Autodesk Fusion 360 part; units mm, degrees
(part 8 of 23)
  arc A626 (13.2203, 51.9113) -> (13.2203, 52.2287) centre (13.2203, 52.07) ccw
  arc A627 (5.1816, 11.4173) -> (5.0292, 11.4173) centre (5.1054, 11.4173) ccw
  line L5 (12.319, 44.069) -> (13.97, 44.069)
  arc A628 (84.2253, 50.6413) -> (84.2253, 50.9588) centre (84.2253, 50.8001) ccw
  arc A629 (10.6803, 51.9113) -> (10.6803, 52.2287) centre (10.6803, 52.07) ccw
  arc A630 (80.3275, 51.5938) -> (80.3275, 51.2763) centre (80.3275, 51.4351) ccw
  line L6 (20.32, 40.64) -> (25.4, 40.64)
  arc A631 (10.1061, 41.9639) -> (10.2139, 41.8561) centre (10.16, 41.91) ccw
  arc A632 (76.9767, 52.5463) -> (76.9767, 52.8638) centre (76.9767, 52.7051) ccw
  arc A633 (25.4, 40.5638) -> (25.4, 40.7162) centre (25.4, 40.64) ccw
  arc A634 (14.7197, 52.2287) -> (14.7197, 51.9113) centre (14.7197, 52.07) ccw
  arc A635 (20.32, 40.7162) -> (20.32, 40.5638) centre (20.32, 40.64) ccw
  arc A636 (4.6355, 51.2763) -> (4.6355, 51.5938) centre (4.6355, 51.4351) ccw
  arc A637 (74.93, 50.9588) -> (74.93, 50.6413) centre (74.93, 50.8001) ccw
  arc A638 (59.7335, 50.6413) -> (59.7335, 50.9588) centre (59.7335, 50.8001) ccw
  arc A639 (17.2597, 52.2287) -> (17.2597, 51.9113) centre (17.2597, 52.07) ccw
  arc A640 (8.0326, 51.5938) -> (8.0326, 51.2763) centre (8.0326, 51.4351) ccw
  arc A641 (22.3397, 52.2287) -> (22.3397, 51.9113) centre (22.3397, 52.07) ccw
  arc A642 (7.9863, 52.8638) -> (7.9863, 52.5463) centre (7.9863, 52.7051) ccw
  arc A643 (4.0005, 51.5938) -> (4.0005, 51.2763) centre (4.0005, 51.4351) ccw
  arc A644 (80.9625, 50.6413) -> (80.9625, 50.9588) centre (80.9625, 50.8001) ccw
  arc A645 (57.1065, 50.9588) -> (57.1065, 50.6413) centre (57.1065, 50.8001) ccw
  arc A646 (23.1009, 51.5938) -> (23.1009, 51.2763) centre (23.1009, 51.4351) ccw
  arc A647 (62.1865, 50.9588) -> (62.1865, 50.6413) centre (62.1865, 50.8001) ccw
  arc A648 (80.3275, 51.9113) -> (80.3275, 52.2287) centre (80.3275, 52.07) ccw
  arc A649 (59.6465, 50.9588) -> (59.6465, 50.6413) centre (59.6465, 50.8001) ccw
  arc A650 (75.5997, 50.9588) -> (75.5997, 50.6413) centre (75.5997, 50.8001) ccw
  arc A651 (19.05, 51.2763) -> (19.05, 51.5938) centre (19.05, 51.4351) ccw
  arc A652 (80.3275, 50.9588) -> (80.3275, 50.6413) centre (80.3275, 50.8001) ccw
  arc A653 (77.0766, 50.6413) -> (77.0766, 50.9588) centre (77.0766, 50.8001) ccw
  arc A654 (57.1935, 50.6413) -> (57.1935, 50.9588) centre (57.1935, 50.8001) ccw
  line L7 (25.4, 40.64) -> (26.67, 41.91)
  line L8 (5.1054, 6.3754) -> (5.1054, 11.4173)
  arc A655 (8.128, 41.9862) -> (8.128, 41.8338) centre (8.128, 41.91) ccw
  arc A656 (71.755, 10.2362) -> (71.755, 10.0838) centre (71.755, 10.16) ccw
  arc A657 (13.9161, 6.2961) -> (14.0239, 6.4039) centre (13.97, 6.35) ccw
  arc A658 (81.0545, 21.3645) -> (80.9467, 21.2567) centre (81.0006, 21.3106) ccw
  arc A659 (80.7212, 21.2344) -> (80.7212, 21.3868) centre (80.7212, 21.3106) ccw
  arc A660 (79.5559, 14.6781) -> (79.4481, 14.7859) centre (79.502, 14.732) ccw
  arc A661 (81.661, 14.6558) -> (81.661, 14.8082) centre (81.661, 14.732) ccw
  arc A662 (12.319, 44.1452) -> (12.319, 43.9928) centre (12.319, 44.069) ccw
  arc A663 (6.088, 55.4038) -> (6.088, 55.0863) centre (6.088, 55.2451) ccw
  arc A664 (5.1593, 6.3215) -> (5.0515, 6.4293) centre (5.1054, 6.3754) ccw
  line L9 (10.16, 41.91) -> (12.319, 44.069)
  arc A665 (26.7462, 38.1) -> (26.5938, 38.1) centre (26.67, 38.1) ccw
  line L10 (82.55, 19.7612) -> (81.0006, 21.3106)
  arc A666 (5.0134, 6.3912) -> (5.1212, 6.2834) centre (5.0673, 6.3373) ccw
  line L11 (5.0673, 6.3373) -> (5.1054, 6.3754)
  arc A667 (78.875, 55.0863) -> (78.875, 55.4038) centre (78.875, 55.2451) ccw
  line L12 (8.128, 41.91) -> (10.16, 41.91)
  arc A668 (82.4738, 15.621) -> (82.6262, 15.621) centre (82.55, 15.621) ccw
  line L13 (5.08, 15.24) -> (7.62, 15.24)
  arc A669 (82.6039, 15.5671) -> (82.4961, 15.6749) centre (82.55, 15.621) ccw
  arc A670 (25.3461, 40.6939) -> (25.4539, 40.5861) centre (25.4, 40.64) ccw
  arc A671 (81.6071, 14.7859) -> (81.7149, 14.6781) centre (81.661, 14.732) ccw
  line L14 (74.2188, 21.3106) -> (80.7212, 21.3106)
  arc A672 (12.3729, 44.0151) -> (12.2651, 44.1229) centre (12.319, 44.069) ccw
  arc A673 (82.4961, 19.7073) -> (82.6039, 19.8151) centre (82.55, 19.7612) ccw
  arc A674 (80.9467, 21.3645) -> (81.0545, 21.2567) centre (81.0006, 21.3106) ccw
  arc A675 (82.6262, 25.4) -> (82.4738, 25.4) centre (82.55, 25.4) ccw
  arc A676 (5.0292, 6.3754) -> (5.1816, 6.3754) centre (5.1054, 6.3754) ccw
  arc A677 (81.0006, 21.2344) -> (81.0006, 21.3868) centre (81.0006, 21.3106) ccw
  arc A678 (13.97, 43.9928) -> (13.97, 44.1452) centre (13.97, 44.069) ccw
  arc A679 (26.5938, 34.29) -> (26.7462, 34.29) centre (26.67, 34.29) ccw
  arc A680 (5.08, 15.3162) -> (5.08, 15.1638) centre (5.08, 15.24) ccw
  line L15 (82.55, 15.621) -> (82.55, 19.7612)
  line L16 (45.72, 17.78) -> (49.53, 13.97)
  arc A681 (11.4839, 8.9439) -> (11.3761, 8.8361) centre (11.43, 8.89) ccw
  arc A682 (82.4738, 22.86) -> (82.6262, 22.86) centre (82.55, 22.86) ccw
  line L17 (41.91, 25.4) -> (41.91, 24.892)
  arc A683 (71.7011, 10.1061) -> (71.8089, 10.2139) centre (71.755, 10.16) ccw
  arc A684 (67.9989, 14.0239) -> (67.8911, 13.9161) centre (67.945, 13.97) ccw
  arc A685 (74.2188, 21.3868) -> (74.2188, 21.2344) centre (74.2188, 21.3106) ccw
  arc A686 (80.7212, 21.3868) -> (80.7212, 21.2344) centre (80.7212, 21.3106) ccw
  arc A687 (82.6262, 19.7612) -> (82.4738, 19.7612) centre (82.55, 19.7612) ccw
  arc A688 (82.6039, 22.8061) -> (82.4961, 22.9139) centre (82.55, 22.86) ccw
  line L18 (81.0006, 21.3106) -> (82.55, 22.86)
  line L19 (74.93, 10.16) -> (79.502, 14.732)
  line L20 (79.502, 14.732) -> (81.661, 14.732)
  arc A689 (11.5062, 11.43) -> (11.3538, 11.43) centre (11.43, 11.43) ccw
  line L21 (7.62, 15.24) -> (11.43, 11.43)
  arc A690 (7.62, 15.1638) -> (7.62, 15.3162) centre (7.62, 15.24) ccw
  arc A691 (45.6438, 17.78) -> (45.7962, 17.78) centre (45.72, 17.78) ccw
  arc A692 (45.7962, 21.082) -> (45.6438, 21.082) centre (45.72, 21.082) ccw
  line L22 (25.4, 49.53) -> (21.59, 49.53)
  line L23 (82.55, 22.86) -> (82.55, 25.4)
  line L24 (49.53, 13.97) -> (67.945, 13.97)
  arc A693 (41.8338, 24.892) -> (41.9862, 24.892) centre (41.91, 24.892) ccw
  line L25 (67.945, 13.97) -> (71.755, 10.16)
  line L26 (11.43, 11.43) -> (11.43, 8.89)
  arc A694 (49.53, 14.0462) -> (49.53, 13.8938) centre (49.53, 13.97) ccw
  arc A695 (74.93, 10.0838) -> (74.93, 10.2362) centre (74.93, 10.16) ccw
  arc A696 (41.9639, 24.9459) -> (41.8561, 24.8381) centre (41.91, 24.892) ccw
  line L27 (11.43, 8.89) -> (13.97, 6.35)
  line L28 (45.72, 21.082) -> (45.72, 17.78)
  arc A697 (25.4, 49.3713) -> (25.4, 49.6887) centre (25.4, 49.53) ccw
  arc A698 (67.945, 13.8938) -> (67.945, 14.0462) centre (67.945, 13.97) ccw
  arc A699 (41.9862, 25.4) -> (41.8338, 25.4) centre (41.91, 25.4) ccw
  arc A700 (7.6739, 15.2939) -> (7.5661, 15.1861) centre (7.62, 15.24) ccw
  arc A701 (45.7739, 17.8339) -> (45.6661, 17.7261) centre (45.72, 17.78) ccw
  arc A702 (49.4761, 13.9161) -> (49.5839, 14.0239) centre (49.53, 13.97) ccw
  line L29 (71.755, 10.16) -> (74.93, 10.16)
  line L30 (45.72, 21.082) -> (41.91, 24.892)
  arc A703 (11.3538, 8.89) -> (11.5062, 8.89) centre (11.43, 8.89) ccw
  line L31 (81.661, 14.732) -> (82.55, 15.621)
  line L32 (80.7212, 21.3106) -> (81.0006, 21.3106)
  line L33 (26.67, 38.1) -> (26.67, 34.29)
  arc A704 (26.7239, 41.8561) -> (26.6161, 41.9639) centre (26.67, 41.91) ccw
  arc A705 (79.502, 14.8082) -> (79.502, 14.6558) centre (79.502, 14.732) ccw
  arc A706 (45.6661, 21.0281) -> (45.7739, 21.1359) centre (45.72, 21.082) ccw
  arc A707 (11.3761, 11.3761) -> (11.4839, 11.4839) centre (11.43, 11.43) ccw
  arc A708 (74.8761, 10.2139) -> (74.9839, 10.1061) centre (74.93, 10.16) ccw
  arc A709 (21.59, 49.6887) -> (21.59, 49.3713) centre (21.59, 49.53) ccw
  arc A710 (57.73, 2.7178) -> (57.73, 2.7686) centre (57.73, 2.7432) ccw
  arc A711 (55.827, 1.5494) -> (55.827, 1.6002) centre (55.827, 1.5748) ccw
  arc A712 (56.3204, 2.7512) -> (56.2722, 2.7352) centre (56.2963, 2.7432) ccw
  arc A713 (54.5067, 2.7178) -> (54.5067, 2.7686) centre (54.5067, 2.7432) ccw
  arc A714 (46.887, 2.4186) -> (46.9378, 2.4186) centre (46.9124, 2.4186) ccw
  arc A715 (59.4219, 1.8994) -> (59.4727, 1.8994) centre (59.4473, 1.8994) ccw
  line L34 (53.2144, 2.0616) -> (53.5715, 2.2564)
  arc A716 (48.3304, 2.0827) -> (48.285, 2.1054) centre (48.3077, 2.0941) ccw
  arc A717 (53.2023, 2.0839) -> (53.2266, 2.0393) centre (53.2145, 2.0616) ccw
  arc A718 (48.6718, 1.5748) -> (48.7226, 1.5748) centre (48.6972, 1.5748) ccw
  line L35 (49.8306, 1.5748) -> (49.8306, 2.7432)
  arc A719 (53.4416, 2.7686) -> (53.4416, 2.7178) centre (53.4416, 2.7432) ccw
  arc A720 (57.73, 1.5494) -> (57.73, 1.6002) centre (57.73, 1.5748) ccw
  arc A721 (58.2535, 2.7432) -> (58.2027, 2.7432) centre (58.2281, 2.7432) ccw
  line L36 (58.8772, 1.5748) -> (58.8772, 2.7432)
  arc A722 (54.8059, 1.5748) -> (54.8567, 1.5748) centre (54.8313, 1.5748) ccw
  arc A723 (55.3077, 2.7686) -> (55.3077, 2.7178) centre (55.3077, 2.7432) ccw
  arc A724 (53.7013, 2.4836) -> (53.4416, 2.7432) centre (53.4416, 2.4835) ccw
  line L37 (55.827, 2.7432) -> (55.3077, 2.7432)
  arc A725 (54.8313, 2.7178) -> (54.8313, 2.7686) centre (54.8313, 2.7432) ccw
  line L38 (54.8313, 1.5748) -> (54.8313, 2.7432)
  arc A726 (49.8052, 1.5748) -> (49.856, 1.5748) centre (49.8306, 1.5748) ccw
  arc A727 (53.6759, 2.4836) -> (53.7267, 2.4836) centre (53.7013, 2.4836) ccw
  arc A728 (59.4727, 2.7432) -> (59.4219, 2.7432) centre (59.4473, 2.7432) ccw
  arc A729 (57.4703, 2.7686) -> (57.4703, 2.7178) centre (57.4703, 2.7432) ccw
  arc A730 (54.5067, 2.7686) -> (54.5067, 2.7178) centre (54.5067, 2.7432) ccw
  arc A731 (46.9124, 1.8994) -> (47.5615, 1.8994) centre (47.237, 1.8994) ccw
  arc A732 (46.9378, 1.8994) -> (46.887, 1.8994) centre (46.9124, 1.8994) ccw
  arc A733 (52.0122, 1.8923) -> (52.0122, 1.8415) centre (52.0122, 1.8669) ccw
  arc A734 (55.827, 2.7178) -> (55.827, 2.7686) centre (55.827, 2.7432) ccw
  arc A735 (53.4416, 2.7432) -> (53.1495, 2.6458) centre (53.4416, 2.2564) ccw
  arc A736 (58.8518, 1.5748) -> (58.9026, 1.5748) centre (58.8772, 1.5748) ccw
  line L39 (54.8313, 2.7432) -> (54.5067, 2.7432)
  arc A737 (54.5067, 2.7432) -> (54.5067, 2.0941) centre (54.5067, 2.4186) ccw
  arc A738 (52.5964, 1.8415) -> (52.5964, 1.8923) centre (52.5964, 1.8669) ccw
  arc A739 (54.5067, 2.0687) -> (54.5067, 2.1195) centre (54.5067, 2.0941) ccw
  arc A740 (49.506, 2.7178) -> (49.506, 2.7686) centre (49.506, 2.7432) ccw
  line L40 (57.6002, 2.7432) -> (57.6002, 1.5748)
  arc A741 (51.8907, 1.5828) -> (51.9389, 1.5668) centre (51.9148, 1.5748) ccw
  arc A742 (53.7518, 1.7192) -> (53.7157, 1.755) centre (53.7338, 1.7371) ccw
  arc A743 (50.9262, 1.6002) -> (50.9262, 1.5494) centre (50.9262, 1.5748) ccw
  line L41 (49.506, 2.0941) -> (49.8306, 2.0941)
  arc A744 (58.8994, 2.7309) -> (58.855, 2.7555) centre (58.8772, 2.7432) ccw
  arc A745 (46.887, 1.8994) -> (46.9378, 1.8994) centre (46.9124, 1.8994) ccw
  arc A746 (49.8306, 2.0687) -> (49.8306, 2.1195) centre (49.8306, 2.0941) ccw
  arc A747 (55.8016, 1.5748) -> (55.8524, 1.5748) centre (55.827, 1.5748) ccw
  line L42 (51.4455, 2.7432) -> (51.4455, 1.5748)
  line L43 (51.4455, 1.5748) -> (50.9262, 1.5748)
  arc A748 (58.2059, 1.5871) -> (58.2503, 1.5625) centre (58.2281, 1.5748) ccw
  arc A749 (53.1343, 2.6662) -> (53.1648, 2.6255) centre (53.1496, 2.6458) ccw
  line L44 (57.73, 2.7432) -> (57.4703, 2.7432)
  arc A750 (57.6256, 2.7432) -> (57.5748, 2.7432) centre (57.6002, 2.7432) ccw
  arc A751 (53.5715, 2.2564) -> (53.7013, 2.4836) centre (53.4376, 2.4836) ccw
  arc A752 (52.3284, 2.7512) -> (52.2802, 2.7352) centre (52.3043, 2.7432) ccw
  arc A753 (49.506, 2.0687) -> (49.506, 2.1195) centre (49.506, 2.0941) ccw
  arc A754 (49.856, 2.7432) -> (49.8052, 2.7432) centre (49.8306, 2.7432) ccw
  arc A755 (48.7226, 2.7432) -> (48.6718, 2.7432) centre (48.6972, 2.7432) ccw
  line L45 (52.6937, 1.5748) -> (52.3043, 2.7432)
  arc A756 (54.8567, 2.7432) -> (54.8059, 2.7432) centre (54.8313, 2.7432) ccw
  arc A757 (48.6972, 2.7178) -> (48.6972, 2.7686) centre (48.6972, 2.7432) ccw
  arc A758 (53.2273, 2.0397) -> (53.2015, 2.0835) centre (53.2144, 2.0616) ccw
  arc A759 (47.5869, 2.4186) -> (47.5361, 2.4186) centre (47.5615, 2.4186) ccw
  arc A760 (49.8306, 2.7178) -> (49.8306, 2.7686) centre (49.8306, 2.7432) ccw
  arc A761 (48.3726, 2.7432) -> (48.3726, 2.0941) centre (48.3726, 2.4186) ccw
  line L46 (48.6972, 2.7432) -> (48.3726, 2.7432)
  line L47 (49.8306, 2.7432) -> (49.506, 2.7432)
  arc A762 (49.506, 2.7686) -> (49.506, 2.7178) centre (49.506, 2.7432) ccw
  arc A763 (48.3726, 2.7178) -> (48.3726, 2.7686) centre (48.3726, 2.7432) ccw
  line L48 (46.9124, 2.4186) -> (46.9124, 1.8994)
  arc A764 (53.2144, 2.0616) -> (53.0846, 1.8344) centre (53.3483, 1.8344) ccw
  arc A765 (53.7267, 2.4836) -> (53.6759, 2.4836) centre (53.7013, 2.4836) ccw
  arc A766 (52.3284, 2.7352) -> (52.2802, 2.7512) centre (52.3043, 2.7432) ccw
  arc A767 (48.0253, 1.5862) -> (48.0708, 1.5634) centre (48.0481, 1.5748) ccw
  line L49 (48.0481, 1.5748) -> (48.3077, 2.0941)
  line L50 (48.6972, 1.5748) -> (48.6972, 2.7432)
  arc A768 (46.9378, 2.4186) -> (46.887, 2.4186) centre (46.9124, 2.4186) ccw
  arc A769 (48.3726, 2.1195) -> (48.3726, 2.0687) centre (48.3726, 2.0941) ccw
  arc A770 (44.3715, 2.7178) -> (44.3715, 2.7686) centre (44.3715, 2.7432) ccw
  arc A771 (43.7515, 2.7178) -> (43.7515, 2.7686) centre (43.7515, 2.7432) ccw
  arc A772 (40.9609, 2.4836) -> (40.9101, 2.4836) centre (40.9355, 2.4836) ccw
  arc A773 (40.4162, 1.6002) -> (40.4162, 1.5494) centre (40.4162, 1.5748) ccw
  arc A774 (41.6956, 2.0687) -> (41.6956, 2.1195) centre (41.6956, 2.0941) ccw
  line L51 (40.9355, 1.8344) -> (40.9355, 2.4836)
  arc A775 (40.9101, 1.8344) -> (40.9609, 1.8344) centre (40.9355, 1.8344) ccw
  arc A776 (47.5615, 2.4186) -> (46.9124, 2.4186) centre (47.237, 2.4186) ccw
  arc A777 (53.5836, 2.2341) -> (53.5593, 2.2787) centre (53.5714, 2.2564) ccw
  line L52 (48.3726, 2.0941) -> (48.6972, 2.0941)
  arc A778 (42.0201, 2.7178) -> (42.0201, 2.7686) centre (42.0201, 2.7432) ccw
  arc A779 (42.0455, 2.7432) -> (41.9947, 2.7432) centre (42.0201, 2.7432) ccw
  arc A780 (48.3726, 2.7686) -> (48.3726, 2.7178) centre (48.3726, 2.7432) ccw
  line L53 (47.5615, 1.8994) -> (47.5615, 2.4186)
  arc A781 (51.4455, 1.5494) -> (51.4455, 1.6002) centre (51.4455, 1.5748) ccw
  arc A782 (47.5361, 2.4186) -> (47.5869, 2.4186) centre (47.5615, 2.4186) ccw
  arc A783 (40.9609, 1.8344) -> (40.9101, 1.8344) centre (40.9355, 1.8344) ccw
  line L54 (45.5781, 2.7432) -> (45.0588, 2.7432)
  arc A784 (46.1458, 1.8344) -> (46.4054, 1.5748) centre (46.4054, 1.8344) ccw
  arc A785 (47.5361, 1.8994) -> (47.5869, 1.8994) centre (47.5615, 1.8994) ccw
  arc A786 (41.6956, 2.7178) -> (41.6956, 2.7686) centre (41.6956, 2.7432) ccw
  arc A787 (45.5781, 2.7178) -> (45.5781, 2.7686) centre (45.5781, 2.7432) ccw
  arc A788 (44.3715, 1.5494) -> (44.3715, 1.6002) centre (44.3715, 1.5748) ccw
  arc A789 (49.506, 2.1195) -> (49.506, 2.0687) centre (49.506, 2.0941) ccw
  arc A790 (44.6566, 2.4836) -> (44.6058, 2.4836) centre (44.6312, 2.4836) ccw
  arc A791 (41.9947, 1.5748) -> (42.0455, 1.5748) centre (42.0201, 1.5748) ccw
  arc A792 (53.4416, 2.7178) -> (53.4416, 2.7686) centre (53.4416, 2.7432) ccw
  arc A793 (51.4709, 2.7432) -> (51.4201, 2.7432) centre (51.4455, 2.7432) ccw
  arc A794 (52.6696, 1.5668) -> (52.7178, 1.5828) centre (52.6937, 1.5748) ccw
  arc A795 (51.4201, 1.5748) -> (51.4709, 1.5748) centre (51.4455, 1.5748) ccw
  line L55 (52.0122, 1.8669) -> (52.5964, 1.8669)
  arc A796 (48.6972, 2.0687) -> (48.6972, 2.1195) centre (48.6972, 2.0941) ccw
  line L56 (52.3043, 2.7432) -> (51.9148, 1.5748)
  arc A797 (53.0592, 1.8344) -> (53.11, 1.8344) centre (53.0846, 1.8344) ccw
  arc A798 (43.4524, 2.7432) -> (43.4016, 2.7432) centre (43.427, 2.7432) ccw
  arc A799 (44.6566, 1.8344) -> (44.6058, 1.8344) centre (44.6312, 1.8344) ccw
  arc A800 (53.5586, 2.2782) -> (53.5843, 2.2345) centre (53.5714, 2.2564) ccw
  arc A801 (46.1204, 1.8344) -> (46.1712, 1.8344) centre (46.1458, 1.8344) ccw
  line L57 (44.6312, 1.8344) -> (44.6312, 2.4836)
  arc A802 (49.506, 2.7432) -> (49.506, 2.0941) centre (49.506, 2.4186) ccw
  arc A803 (45.0588, 2.7686) -> (45.0588, 2.7178) centre (45.0588, 2.7432) ccw
  arc A804 (45.5781, 1.5494) -> (45.5781, 1.6002) centre (45.5781, 1.5748) ccw
  arc A805 (48.3726, 2.0687) -> (48.3726, 2.1195) centre (48.3726, 2.0941) ccw
  line L58 (42.0201, 1.5748) -> (42.0201, 2.7432)
  arc A806 (44.6058, 2.4836) -> (44.6566, 2.4836) centre (44.6312, 2.4836) ccw
  line L59 (45.5781, 2.2239) -> (45.1886, 2.2239)
  line L60 (40.4162, 1.5748) -> (40.6758, 1.5748)
  arc A807 (43.4016, 1.5748) -> (43.4524, 1.5748) centre (43.427, 1.5748) ccw
  arc A808 (36.7595, 1.5494) -> (36.7595, 1.6002) centre (36.7595, 1.5748) ccw
  arc A809 (36.6946, 2.7432) -> (36.6946, 2.2239) centre (36.6946, 2.4836) ccw
  arc A810 (44.1119, 1.6002) -> (44.1119, 1.5494) centre (44.1119, 1.5748) ccw
  arc A811 (40.9355, 2.4836) -> (40.6758, 2.7432) centre (40.6758, 2.4835) ccw
  arc A812 (46.5352, 1.5494) -> (46.5352, 1.6002) centre (46.5352, 1.5748) ccw
  arc A813 (39.6001, 2.1985) -> (39.6001, 2.2493) centre (39.6001, 2.2239) ccw
  arc A814 (36.6946, 2.7178) -> (36.6946, 2.7686) centre (36.6946, 2.7432) ccw
  arc A815 (39.6001, 2.1985) -> (39.6001, 2.2493) centre (39.6001, 2.2239) ccw
  arc A816 (40.6758, 1.6002) -> (40.6758, 1.5494) centre (40.6758, 1.5748) ccw
  line L61 (45.0588, 1.5748) -> (45.5781, 1.5748)
  arc A817 (43.1024, 2.7686) -> (43.1024, 2.7178) centre (43.1024, 2.7432) ccw
  arc A818 (45.5527, 1.5748) -> (45.6035, 1.5748) centre (45.5781, 1.5748) ccw
  arc A819 (39.9246, 2.7178) -> (39.9246, 2.7686) centre (39.9246, 2.7432) ccw
  arc A820 (37.084, 1.5494) -> (37.084, 1.6002) centre (37.084, 1.5748) ccw
  line L62 (41.6956, 2.0941) -> (42.0201, 2.0941)
  arc A821 (41.6956, 2.1195) -> (41.6956, 2.0687) centre (41.6956, 2.0941) ccw
  arc A822 (46.1712, 1.8344) -> (46.1204, 1.8344) centre (46.1458, 1.8344) ccw
  arc A823 (41.6956, 2.7432) -> (41.6956, 2.0941) centre (41.6956, 2.4186) ccw
  arc A824 (39.6001, 1.6002) -> (39.6001, 1.5494) centre (39.6001, 1.5748) ccw
  arc A825 (41.6956, 2.7686) -> (41.6956, 2.7178) centre (41.6956, 2.7432) ccw
  line L63 (46.4054, 1.5748) -> (46.5352, 1.5748)
  arc A826 (46.4054, 1.5494) -> (46.4054, 1.6002) centre (46.4054, 1.5748) ccw
  line L64 (43.7515, 2.7432) -> (43.1024, 2.7432)
  line L65 (44.1119, 1.5748) -> (44.3715, 1.5748)
  arc A827 (40.4162, 2.7686) -> (40.4162, 2.7178) centre (40.4162, 2.7432) ccw
  arc A828 (44.6312, 2.4836) -> (44.3715, 2.7432) centre (44.3715, 2.4835) ccw
  arc A829 (46.4054, 1.6002) -> (46.4054, 1.5494) centre (46.4054, 1.5748) ccw
  arc A830 (40.9101, 2.4836) -> (40.9609, 2.4836) centre (40.9355, 2.4836) ccw
  arc A831 (36.6946, 2.1985) -> (36.6946, 2.2493) centre (36.6946, 2.2239) ccw
  arc A832 (45.1886, 2.2493) -> (45.1886, 2.1985) centre (45.1886, 2.2239) ccw
  line L66 (46.1458, 2.7432) -> (46.1458, 1.8344)
  arc A833 (44.3715, 1.5748) -> (44.6312, 1.8344) centre (44.3715, 1.8345) ccw
  arc A834 (45.0588, 1.6002) -> (45.0588, 1.5494) centre (45.0588, 1.5748) ccw
  line L67 (44.3715, 2.7432) -> (44.1119, 2.7432)
  line L68 (45.5781, 1.5748) -> (45.5781, 2.7432)
  arc A835 (45.5781, 2.1985) -> (45.5781, 2.2493) centre (45.5781, 2.2239) ccw
  arc A836 (39.6001, 2.2239) -> (39.6001, 1.5748) centre (39.6001, 1.8994) ccw
  arc A837 (44.3715, 2.7686) -> (44.3715, 2.7178) centre (44.3715, 2.7432) ccw
  arc A838 (44.6058, 1.8344) -> (44.6566, 1.8344) centre (44.6312, 1.8344) ccw
  line L69 (37.9025, 1.5748) -> (37.513, 2.7432)
  arc A839 (36.9542, 2.1985) -> (36.9542, 2.2493) centre (36.9542, 2.2239) ccw
  arc A840 (36.6946, 2.7686) -> (36.6946, 2.7178) centre (36.6946, 2.7432) ccw
  line L70 (39.9246, 1.5748) -> (39.9246, 2.7432)
  arc A841 (40.6758, 2.7686) -> (40.6758, 2.7178) centre (40.6758, 2.7432) ccw
  arc A842 (42.0201, 2.0687) -> (42.0201, 2.1195) centre (42.0201, 2.0941) ccw
  line L71 (42.0201, 2.7432) -> (41.6956, 2.7432)
  arc A843 (38.3161, 2.7352) -> (38.2679, 2.7512) centre (38.292, 2.7432) ccw
  arc A844 (47.5869, 1.8994) -> (47.5361, 1.8994) centre (47.5615, 1.8994) ccw
  arc A845 (45.6035, 2.7432) -> (45.5527, 2.7432) centre (45.5781, 2.7432) ccw
  arc A846 (40.6758, 1.5748) -> (40.9355, 1.8344) centre (40.6758, 1.8345) ccw
  arc A847 (44.3715, 1.6002) -> (44.3715, 1.5494) centre (44.3715, 1.5748) ccw
  arc A848 (40.6758, 1.5494) -> (40.6758, 1.6002) centre (40.6758, 1.5748) ccw
  line L72 (43.427, 1.5748) -> (43.427, 2.7432)
  arc A849 (46.1712, 2.7432) -> (46.1204, 2.7432) centre (46.1458, 2.7432) ccw
  arc A850 (44.1119, 2.7686) -> (44.1119, 2.7178) centre (44.1119, 2.7432) ccw
  arc A851 (39.6001, 2.7178) -> (39.6001, 2.7686) centre (39.6001, 2.7432) ccw
  arc A852 (39.6001, 1.5494) -> (39.6001, 1.6002) centre (39.6001, 1.5748) ccw
  arc A853 (48.8132, 13.5283) -> (48.5887, 13.3038) centre (48.701, 13.416) ccw
  arc A854 (43.3224, 25.6494) -> (43.0049, 25.6494) centre (43.1637, 25.6494) ccw
  line L73 (40.8472, 24.6898) -> (40.9976, 24.5394)
  arc A855 (39.6001, 2.2493) -> (39.6001, 2.1985) centre (39.6001, 2.2239) ccw
  arc A856 (48.8638, 13.0287) -> (49.0883, 13.2532) centre (48.9761, 13.1409) ccw
  arc A857 (42.7324, 26.5751) -> (42.5079, 26.3506) centre (42.6201, 26.4629) ccw
  arc A858 (44.6298, 20.5647) -> (44.8544, 20.7892) centre (44.7421, 20.677) ccw
  line L74 (40.8472, 26.1102) -> (40.6563, 25.6494)
  arc A859 (39.9246, 1.5494) -> (39.9246, 1.6002) centre (39.9246, 1.5748) ccw
  arc A860 (37.084, 2.7178) -> (37.084, 2.7686) centre (37.084, 2.7432) ccw
  arc A861 (49.2747, 12.8454) -> (49.3962, 13.1388) centre (49.3355, 12.9921) ccw
  arc A862 (40.9594, 24.8021) -> (40.7349, 24.5776) centre (40.8472, 24.6898) ccw
  line L75 (48.701, 13.4161) -> (48.9761, 13.141)
  arc A863 (42.2201, 26.8004) -> (42.0986, 26.507) centre (42.1594, 26.6537) ccw
  arc A864 (42.5594, 26.3162) -> (42.6809, 26.6095) centre (42.6201, 26.4628) ccw
  line L76 (39.9246, 2.7432) -> (39.6001, 2.7432)
  line L77 (38.292, 2.7432) -> (37.9025, 1.5748)
  arc A865 (40.6758, 2.7178) -> (40.6758, 2.7686) centre (40.6758, 2.7432) ccw
  line L78 (37.084, 2.7432) -> (36.6946, 2.7432)
  arc A866 (39.8992, 1.5748) -> (39.95, 1.5748) centre (39.9246, 1.5748) ccw
  line L79 (40.6758, 2.7432) -> (40.4162, 2.7432)
  line L80 (44.7421, 20.6769) -> (44.7421, 17.5855)
  line L81 (12.3063, 34.2399) -> (12.3063, 33.5781)
  line L82 (37.084, 1.5748) -> (36.7595, 1.5748)
  line L83 (36.6946, 2.2239) -> (36.9542, 2.2239)
  arc A867 (41.1391, 26.6095) -> (41.2606, 26.3162) centre (41.1998, 26.4628) ccw
  arc A868 (41.3121, 26.3506) -> (41.0876, 26.5751) centre (41.1998, 26.4629) ccw
  line L84 (40.9976, 24.5394) -> (41.081, 24.3381)
  line L85 (39.9246, 2.2239) -> (39.6001, 2.2239)
  arc A869 (36.7595, 2.1985) -> (36.7595, 2.2493) centre (36.7595, 2.2239) ccw
  arc A870 (36.7595, 1.6002) -> (36.7595, 1.5494) centre (36.7595, 1.5748) ccw
  arc A871 (41.1442, 24.6002) -> (40.8509, 24.4787) centre (40.9976, 24.5395) ccw
  arc A872 (36.6946, 2.2493) -> (36.6946, 2.1985) centre (36.6946, 2.2239) ccw
  arc A873 (37.8784, 1.5828) -> (37.9266, 1.5668) centre (37.9025, 1.5748) ccw
  line L86 (41.1998, 26.4628) -> (40.8472, 26.1102)
  line L87 (40.6563, 25.1506) -> (40.8472, 24.6898)
  arc A874 (42.8606, 25.9979) -> (43.0851, 26.2224) centre (42.9729, 26.1102) ccw
  arc A875 (37.8784, 1.5668) -> (37.9266, 1.5828) centre (37.9025, 1.5748) ccw
  arc A876 (40.9938, 26.0494) -> (40.7005, 26.1709) centre (40.8471, 26.1102) ccw
  arc A877 (40.803, 25.2114) -> (40.5096, 25.0899) centre (40.6563, 25.1506) ccw
  arc A878 (36.7595, 2.2239) -> (36.7595, 1.5748) centre (36.7595, 1.8994) ccw
  line L88 (39.6001, 1.5748) -> (39.9246, 1.5748)
  arc A879 (48.5887, 13.3038) -> (48.8132, 13.5283) centre (48.701, 13.416) ccw
  line L89 (48.9761, 13.141) -> (49.3355, 12.9921)
  arc A880 (40.8853, 24.4272) -> (41.1098, 24.6517) centre (40.9976, 24.5395) ccw
  arc A881 (39.95, 2.7432) -> (39.8992, 2.7432) centre (39.9246, 2.7432) ccw
  arc A882 (39.9246, 2.1985) -> (39.9246, 2.2493) centre (39.9246, 2.2239) ccw
  line L90 (43.1637, 25.6494) -> (42.9728, 26.1102)
  line L91 (41.081, 24.3381) -> (41.3561, 24.063)
  arc A883 (39.6001, 2.7432) -> (39.6001, 2.2239) centre (39.6001, 2.4836) ccw
  line L92 (44.891, 17.2261) -> (48.701, 13.4161)
  arc A884 (39.6001, 2.7686) -> (39.6001, 2.7178) centre (39.6001, 2.7432) ccw
  arc A885 (43.3104, 25.0899) -> (43.017, 25.2114) centre (43.1637, 25.1507) ccw
  line L93 (44.7421, 17.5855) -> (44.891, 17.2261)
  arc A886 (37.5371, 2.7512) -> (37.4889, 2.7352) centre (37.513, 2.7432) ccw
  arc A887 (45.0032, 17.3383) -> (44.7787, 17.1138) centre (44.891, 17.226) ccw
  line L94 (43.1258, 25.0591) -> (43.1637, 25.1506)
  arc A888 (46.1617, 21.7988) -> (46.3862, 22.0233) centre (46.2739, 21.9111) ccw
  line L95 (42.6202, 26.4628) -> (42.1594, 26.6537)
  arc A889 (41.6606, 26.8124) -> (41.6606, 26.4949) centre (41.6606, 26.6536) ccw
  arc A890 (43.0049, 25.1506) -> (43.3224, 25.1506) centre (43.1637, 25.1506) ccw
  arc A891 (41.4683, 24.1752) -> (41.2438, 23.9507) centre (41.356, 24.063) ccw
  arc A892 (79.2435, 8.2232) -> (79.2435, 8.5407) centre (79.2435, 8.3819) ccw
  arc A893 (40.4976, 25.1506) -> (40.815, 25.1506) centre (40.6563, 25.1506) ccw
  arc A894 (42.9791, 25.1199) -> (43.2725, 24.9984) centre (43.1258, 25.0592) ccw
  arc A895 (41.2438, 23.9507) -> (41.4683, 24.1752) centre (41.356, 24.063) ccw
  line L96 (79.2435, 8.382) -> (75.7524, 8.382)
  line L97 (71.5605, 9.1821) -> (75.1245, 9.1821)
  arc A896 (44.5834, 17.5855) -> (44.9008, 17.5855) centre (44.7421, 17.5855) ccw
  line L98 (40.6563, 25.6494) -> (40.6563, 25.1506)
  arc A897 (43.017, 25.5886) -> (43.3104, 25.7101) centre (43.1637, 25.6493) ccw
  arc A898 (44.7443, 17.1653) -> (45.0376, 17.2868) centre (44.891, 17.226) ccw
  arc A899 (42.1594, 26.4949) -> (42.1594, 26.8124) centre (42.1594, 26.6536) ccw
  line L99 (81.1911, 11.8305) -> (81.6991, 11.3225)
  line L100 (41.3561, 24.063) -> (44.7421, 20.6769)
  arc A900 (81.1003, 9.0106) -> (81.1003, 9.3281) centre (81.1003, 9.1694) ccw
  arc A901 (80.4587, 9.0227) -> (80.3372, 9.3161) centre (80.398, 9.1694) ccw
  line L101 (49.3355, 12.9921) -> (67.5399, 12.9921)
  arc A902 (81.5404, 9.737) -> (81.8578, 9.737) centre (81.6991, 9.737) ccw
  arc A903 (81.8555, 13.5954) -> (81.8555, 13.9129) centre (81.8555, 13.7542) ccw
  arc A904 (81.0101, 9.2725) -> (81.2346, 9.048) centre (81.1223, 9.1603) ccw
  line L102 (70.926, 9.6061) -> (71.2011, 9.331)
  arc A905 (68.8686, 22.0663) -> (68.8686, 22.3838) centre (68.8686, 22.2251) ccw
  line L103 (42.9728, 26.1102) -> (42.6202, 26.4628)
  arc A906 (43.1195, 26.1709) -> (42.8262, 26.0494) centre (42.9729, 26.1102) ccw
  arc A907 (81.0324, 11.8305) -> (81.3499, 11.8305) centre (81.1912, 11.8305) ccw
  line L104 (79.7492, 8.9006) -> (79.2526, 8.4041)
  line L105 (41.6606, 26.6537) -> (41.1998, 26.4628)
  line L106 (43.1637, 25.1506) -> (43.1637, 25.6494)
  arc A908 (81.0616, 9.0136) -> (81.1831, 9.3069) centre (81.1223, 9.1602) ccw
  line L107 (81.9037, 13.7741) -> (81.1911, 13.0615)
  line L108 (42.1594, 26.6537) -> (41.6606, 26.6537)
  arc A909 (75.6058, 8.3213) -> (75.8991, 8.4427) centre (75.7525, 8.382) ccw
  arc A910 (75.3717, 9.4432) -> (75.5962, 9.2187) centre (75.484, 9.331) ccw
  arc A911 (40.7349, 26.2224) -> (40.9594, 25.9979) centre (40.8472, 26.1102) ccw
  line L109 (81.6991, 9.737) -> (81.1223, 9.1603)
  arc A912 (71.0382, 9.7183) -> (70.8137, 9.4938) centre (70.926, 9.606) ccw
  line L110 (67.5399, 12.9921) -> (70.926, 9.6061)
  arc A913 (79.1403, 8.5163) -> (79.3648, 8.2918) centre (79.2525, 8.4041) ccw
  arc A914 (82.0159, 13.6618) -> (81.7914, 13.8863) centre (81.9036, 13.774) ccw
  arc A915 (40.7005, 24.6291) -> (40.9938, 24.7506) centre (40.8471, 24.6898) ccw
  arc A916 (40.9343, 24.2773) -> (41.2276, 24.3988) centre (41.081, 24.3381) ccw
  arc A917 (44.8888, 17.6462) -> (44.5954, 17.5247) centre (44.7421, 17.5855) ccw
  arc A918 (41.7214, 26.507) -> (41.5999, 26.8004) centre (41.6606, 26.6537) ccw
  arc A919 (40.815, 25.6494) -> (40.4976, 25.6494) centre (40.6563, 25.6494) ccw
  arc A920 (41.1932, 24.4503) -> (40.9687, 24.2258) centre (41.081, 24.338) ccw
  line L111 (75.4839, 9.331) -> (79.9071, 13.7541)
  line L112 (75.7524, 8.382) -> (75.7433, 8.4041)
  arc A921 (80.0193, 13.6418) -> (79.7948, 13.8664) centre (79.907, 13.7541) ccw
  arc A922 (40.5096, 25.7101) -> (40.803, 25.5886) centre (40.6563, 25.6494) ccw
  line L113 (80.398, 9.1694) -> (79.7492, 8.9006)
  arc A923 (80.398, 9.3281) -> (80.398, 9.0106) centre (80.398, 9.1694) ccw
  arc A924 (44.9008, 20.6769) -> (44.5834, 20.6769) centre (44.7421, 20.6769) ccw
  arc A925 (67.5399, 12.8334) -> (67.5399, 13.1509) centre (67.5399, 12.9922) ccw
  line L114 (79.2526, 8.4041) -> (79.2435, 8.382)
  arc A926 (43.2381, 25.1714) -> (43.0136, 24.9469) centre (43.1258, 25.0591) ccw
  arc A927 (67.6522, 13.1044) -> (67.4277, 12.8798) centre (67.5399, 12.9921) ccw
  arc A928 (71.0888, 9.2187) -> (71.3133, 9.4432) centre (71.2011, 9.331) ccw
  line L115 (71.2011, 9.331) -> (71.5605, 9.1821)
  arc A929 (81.1611, 9.3161) -> (81.0395, 9.0227) centre (81.1003, 9.1694) ccw
  arc A930 (66.1005, 9.3891) -> (66.3938, 9.5106) centre (66.2472, 9.4498) ccw
  line L116 (81.1223, 9.1603) -> (81.1003, 9.1694)
  arc A931 (66.9999, 8.7596) -> (67.1214, 9.053) centre (67.0606, 8.9063) ccw
  line L117 (81.8555, 13.7541) -> (81.9037, 13.7741)
  line L118 (67.5594, 8.9063) -> (68.0202, 9.0972)
  arc A932 (79.0968, 8.4427) -> (79.3901, 8.3213) centre (79.2435, 8.382) ccw
  arc A933 (73.9563, 9.0227) -> (73.8348, 9.3161) centre (73.8956, 9.1694) ccw
  line L119 (68.0202, 11.2228) -> (67.5594, 11.4137)
  arc A934 (72.5944, 8.4427) -> (72.8877, 8.3213) centre (72.7411, 8.382) ccw
  line L120 (75.7433, 8.4041) -> (75.2467, 8.9006)
  arc A935 (70.8137, 9.4938) -> (71.0382, 9.7183) centre (70.926, 9.6061) ccw
  arc A936 (49.3355, 13.1509) -> (49.3355, 12.8334) centre (49.3355, 12.9922) ccw
  arc A937 (71.4997, 9.0354) -> (71.6212, 9.3288) centre (71.5605, 9.1821) ccw
  arc A938 (75.1859, 8.754) -> (75.3075, 9.0473) centre (75.2467, 8.9007) ccw
  arc A939 (75.359, 9.0129) -> (75.1344, 8.7884) centre (75.2467, 8.9006) ccw
  line L121 (75.2467, 8.9006) -> (74.5979, 9.1694)
  line L122 (66.5998, 11.2228) -> (66.2472, 10.8702)
  line L123 (66.0563, 10.4094) -> (66.0563, 9.9106)
  arc A940 (81.8114, 9.6248) -> (81.5868, 9.8493) centre (81.6991, 9.737) ccw
  arc A941 (79.6884, 9.0473) -> (79.8099, 8.754) centre (79.7492, 8.9007) ccw
  arc A942 (75.7524, 8.5407) -> (75.7524, 8.2232) centre (75.7524, 8.3819) ccw
  arc A943 (75.0638, 9.3288) -> (75.1853, 9.0354) centre (75.1245, 9.1821) ccw
  arc A944 (65.8976, 9.9106) -> (66.2151, 9.9106) centre (66.0564, 9.9106) ccw
  line L124 (79.9071, 13.7541) -> (81.8555, 13.7541)
  arc A945 (71.5605, 9.3408) -> (71.5605, 9.0234) centre (71.5605, 9.1821) ccw
  line L125 (81.1911, 13.0615) -> (81.1911, 11.8305)
  arc A946 (81.3499, 13.0615) -> (81.0324, 13.0615) centre (81.1912, 13.0615) ccw
  arc A947 (67.1214, 11.267) -> (66.9999, 11.5604) centre (67.0606, 11.4137) ccw
  arc A948 (81.7948, 13.9008) -> (81.9163, 13.6074) centre (81.8556, 13.7541) ccw
  arc A949 (81.5868, 11.2103) -> (81.8114, 11.4348) centre (81.6991, 11.3225) ccw
  line L126 (69.1454, 11.1379) -> (68.1051, 11.1379)
  arc A950 (66.2151, 10.4094) -> (65.8976, 10.4094) centre (66.0564, 10.4094) ccw
  arc A951 (72.8969, 8.3433) -> (72.6035, 8.4648) centre (72.7502, 8.4041) ccw
  line L127 (75.1245, 9.1821) -> (75.4839, 9.331)
  arc A952 (79.3993, 8.3433) -> (79.1059, 8.4648) centre (79.2526, 8.4041) ccw
  arc A953 (75.89, 8.4648) -> (75.5966, 8.3433) centre (75.7433, 8.4041) ccw
  arc A954 (71.2618, 9.4776) -> (71.1403, 9.1843) centre (71.201, 9.3309) ccw
  arc A955 (81.8578, 11.3225) -> (81.5404, 11.3225) centre (81.6991, 11.3225) ccw
  arc A956 (67.6201, 11.5604) -> (67.4986, 11.267) centre (67.5593, 11.4137) ccw
  arc A957 (49.0368, 13.2876) -> (48.9153, 12.9943) centre (48.9761, 13.141) ccw
  line L128 (81.1003, 9.1694) -> (80.398, 9.1694)
  line L129 (81.6991, 11.3225) -> (81.6991, 9.737)
  arc A958 (67.5594, 8.7476) -> (67.5594, 9.065) centre (67.5594, 8.9063) ccw
  arc A959 (67.0606, 9.065) -> (67.0606, 8.7476) centre (67.0606, 8.9063) ccw
  line L130 (69.5048, 10.989) -> (69.1454, 11.1379)
  arc A960 (74.6586, 9.3161) -> (74.5371, 9.0227) centre (74.5978, 9.1694) ccw
  arc A961 (79.8614, 8.7884) -> (79.6369, 9.0129) centre (79.7491, 8.9006) ccw
  line L131 (67.0606, 8.9063) -> (67.5594, 8.9063)
  arc A962 (69.1454, 10.9791) -> (69.1454, 11.2966) centre (69.1454, 11.1379) ccw
  arc A963 (81.9644, 13.6274) -> (81.8429, 13.9207) centre (81.9037, 13.7741) ccw
  arc A964 (75.1245, 9.0234) -> (75.1245, 9.3408) centre (75.1245, 9.1821) ccw
  arc A965 (75.5447, 9.1843) -> (75.4232, 9.4776) centre (75.484, 9.331) ccw
  arc A966 (79.9071, 13.9129) -> (79.9071, 13.5954) centre (79.9071, 13.7542) ccw
  arc A967 (81.3034, 11.9428) -> (81.0788, 11.7183) centre (81.1911, 11.8306) ccw
  arc A968 (66.5391, 11.3695) -> (66.6606, 11.0762) centre (66.5999, 11.2229) ccw
  arc A969 (81.0788, 13.1737) -> (81.3034, 12.9492) centre (81.1911, 13.0615) ccw
  arc A970 (72.7411, 8.2232) -> (72.7411, 8.5407) centre (72.7411, 8.3819) ccw
  arc A971 (69.617, 11.1013) -> (69.3925, 10.8768) centre (69.5048, 10.989) ccw
  arc A972 (66.203, 9.9714) -> (65.9096, 9.8499) centre (66.0563, 9.9107) ccw
  arc A973 (68.1051, 11.2966) -> (68.1051, 10.9791) centre (68.1051, 11.1379) ccw
  arc A974 (69.2061, 11.2846) -> (69.0846, 10.9912) centre (69.1454, 11.1379) ccw
  arc A975 (67.9594, 11.0762) -> (68.0809, 11.3695) centre (68.0202, 11.2228) ccw
  arc A976 (71.9995, 8.2697) -> (72.2241, 8.4943) centre (72.1118, 8.382) ccw
  line L132 (66.5998, 9.0972) -> (67.0606, 8.9063)
  arc A977 (73.186, 9.0473) -> (73.3075, 8.754) centre (73.2468, 8.9007) ccw
  line L133 (68.1051, 11.1379) -> (68.0202, 11.2228)
  arc A978 (67.9079, 9.2094) -> (68.1324, 8.9849) centre (68.0202, 9.0971) ccw
  line L134 (72.7502, 8.4041) -> (72.7411, 8.382)
  line L135 (67.5594, 11.4137) -> (67.0606, 11.4137)
  arc A979 (72.7411, 6.2675) -> (72.7411, 6.585) centre (72.7411, 6.4263) ccw
  arc A980 (79.2435, 6.2675) -> (79.2435, 6.585) centre (79.2435, 6.4263) ccw
  arc A981 (80.3372, 5.4921) -> (80.4587, 5.7855) centre (80.398, 5.6388) ccw
  arc A982 (75.3075, 5.7609) -> (75.1859, 6.0542) centre (75.2467, 5.9076) ccw
  arc A983 (81.6368, 6.0198) -> (81.8614, 5.7953) centre (81.7491, 5.9075) ccw
  arc A984 (72.1118, 8.5407) -> (72.1118, 8.2232) centre (72.1118, 8.3819) ccw
  arc A985 (66.7121, 11.1106) -> (66.4876, 11.3351) centre (66.5999, 11.2228) ccw
  line L136 (74.5979, 9.1694) -> (73.8956, 9.1694)
  arc A986 (66.3938, 10.8094) -> (66.1005, 10.9309) centre (66.2472, 10.8702) ccw
  arc A987 (65.9096, 10.4701) -> (66.203, 10.3486) centre (66.0563, 10.4093) ccw
  arc A988 (74.5979, 5.4801) -> (74.5979, 5.7976) centre (74.5979, 5.6389) ccw
  arc A989 (67.9928, 11.0256) -> (68.2174, 11.2502) centre (68.1051, 11.1379) ccw
  arc A990 (66.3594, 9.5621) -> (66.1349, 9.3376) centre (66.2472, 9.4498) ccw
  line L137 (67.0606, 11.4137) -> (66.5998, 11.2228)
  arc A991 (68.1324, 11.3351) -> (67.9079, 11.1106) centre (68.0202, 11.2228) ccw
  arc A992 (66.1349, 10.9824) -> (66.3594, 10.7579) centre (66.2472, 10.8702) ccw
  line L138 (73.8956, 9.1694) -> (73.2468, 8.9006)
  arc A993 (69.444, 10.8424) -> (69.5655, 11.1357) centre (69.5048, 10.989) ccw
  arc A994 (73.359, 8.7884) -> (73.1345, 9.0129) centre (73.2468, 8.9006) ccw
  line L139 (66.0563, 9.9106) -> (66.2472, 9.4498)
  arc A995 (66.6606, 9.2438) -> (66.5391, 8.9505) centre (66.5999, 9.0972) ccw
  line L140 (79.2435, 6.4262) -> (79.2526, 6.4041)
  line L141 (68.5458, 9.1821) -> (70.8777, 6.8502)
  arc A996 (79.3901, 6.4869) -> (79.0968, 6.3655) centre (79.2435, 6.4262) ccw
  line L142 (75.7433, 6.4041) -> (75.7524, 6.4262)
  line L143 (82.2457, 6.4041) -> (82.5144, 7.053)
  arc A997 (74.5979, 9.0106) -> (74.5979, 9.3281) centre (74.5979, 9.1694) ccw
  line L144 (75.7524, 6.4262) -> (79.2435, 6.4262)
  line L145 (73.2468, 8.9006) -> (72.7502, 8.4041)
  arc A998 (73.8956, 9.3281) -> (73.8956, 9.0106) centre (73.8956, 9.1694) ccw
  line L146 (66.2472, 9.4498) -> (66.5998, 9.0972)
  arc A999 (66.4876, 8.9849) -> (66.7121, 9.2094) centre (66.5999, 9.0972) ccw
  line L147 (72.7411, 8.382) -> (72.1118, 8.382)
  arc A1000 (67.0606, 11.5724) -> (67.0606, 11.2549) centre (67.0606, 11.4137) ccw
  arc A1001 (75.631, 8.2918) -> (75.8555, 8.5163) centre (75.7433, 8.4041) ccw
  line L148 (66.2472, 10.8702) -> (66.0563, 10.4094)
  line L149 (72.1118, 8.382) -> (69.5048, 10.989)
  arc A1002 (67.5594, 11.2549) -> (67.5594, 11.5724) centre (67.5594, 11.4137) ccw
  arc A1003 (79.8099, 6.0542) -> (79.6884, 5.7609) centre (79.7492, 5.9076) ccw
  arc A1004 (72.6379, 8.5163) -> (72.8624, 8.2918) centre (72.7501, 8.4041) ccw
  line L150 (81.7491, 5.9076) -> (82.2457, 6.4041)
  arc A1005 (71.0405, 6.4628) -> (71.2651, 6.6873) centre (71.1528, 6.5751) ccw
  line L151 (79.7492, 5.9076) -> (80.398, 5.6388)
  arc A1006 (72.6035, 6.3434) -> (72.8969, 6.4649) centre (72.7502, 6.4042) ccw
  arc A1007 (81.1003, 5.4801) -> (81.1003, 5.7976) centre (81.1003, 5.6389) ccw
  arc A1008 (70.99, 6.9624) -> (70.7655, 6.7379) centre (70.8778, 6.8501) ccw
  arc A1009 (68.5458, 9.0234) -> (68.5458, 9.3408) centre (68.5458, 9.1821) ccw
  arc A1010 (75.8555, 6.2919) -> (75.631, 6.5164) centre (75.7433, 6.4041) ccw
  arc A1011 (67.4986, 9.053) -> (67.6201, 8.7596) centre (67.5593, 8.9063) ccw
  line L152 (80.398, 5.6388) -> (81.1003, 5.6388)
  line L153 (70.8777, 6.8502) -> (71.1528, 6.5751)
  arc A1012 (79.6369, 5.7953) -> (79.8614, 6.0198) centre (79.7491, 5.9076) ccw
  arc A1013 (71.2136, 6.7217) -> (71.0921, 6.4284) centre (71.1529, 6.5751) ccw
  line L154 (68.1051, 9.1821) -> (68.5458, 9.1821)
  line L155 (68.0202, 9.0972) -> (68.1051, 9.1821)
  line L156 (72.7411, 6.4262) -> (72.7502, 6.4041)
  line L157 (81.1003, 5.6388) -> (81.7491, 5.9076)
  line L158 (71.1528, 6.5751) -> (71.5122, 6.4262)
  arc A1014 (81.0395, 5.7855) -> (81.161, 5.4921) centre (81.1003, 5.6388) ccw
  line L159 (1.1279, 35.1317) -> (0.9017, 34.5856)
  arc A1015 (74.5371, 5.7855) -> (74.6586, 5.4921) centre (74.5978, 5.6388) ccw
  arc A1016 (60.0182, 19.5923) -> (59.7936, 19.8168) centre (59.9059, 19.7046) ccw
  arc A1017 (59.7936, 20.8232) -> (60.0182, 21.0477) centre (59.9059, 20.9355) ccw
  line L160 (0.9017, 34.5856) -> (0.9017, 33.9944)
  arc A1018 (1.0605, 34.5856) -> (0.7429, 34.5856) centre (0.9017, 34.5856) ccw
  line L161 (0.9017, 33.9944) -> (1.1279, 33.4483)
  arc A1019 (68.658, 9.2944) -> (68.4335, 9.0698) centre (68.5457, 9.1821) ccw
  line L162 (74.5979, 5.6388) -> (75.2467, 5.9076)
  arc A1020 (72.8624, 6.5164) -> (72.6379, 6.2919) centre (72.7501, 6.4041) ccw
  arc A1021 (68.0809, 8.9505) -> (67.9594, 9.2438) centre (68.0202, 9.0972) ccw
  arc A1022 (73.1345, 5.7953) -> (73.359, 6.0198) centre (73.2468, 5.9076) ccw
  arc A1023 (72.8877, 6.4869) -> (72.5944, 6.3655) centre (72.7411, 6.4262) ccw
  arc A1024 (68.2174, 9.0698) -> (67.9928, 9.2944) centre (68.1051, 9.1821) ccw
  line L163 (73.2468, 5.9076) -> (73.8956, 5.6388)
  arc A1025 (70.7655, 6.7379) -> (70.99, 6.9624) centre (70.8778, 6.8502) ccw
  line L164 (75.2467, 5.9076) -> (75.7433, 6.4041)
  arc A1026 (75.8991, 6.3655) -> (75.6058, 6.4869) centre (75.7525, 6.4262) ccw
  arc A1027 (82.3579, 6.2919) -> (82.1334, 6.5164) centre (82.2456, 6.4041) ccw
  line L165 (79.2526, 6.4041) -> (79.7492, 5.9076)
  arc A1028 (79.3648, 6.5164) -> (79.1403, 6.2919) centre (79.2525, 6.4042) ccw
  arc A1029 (71.5122, 6.585) -> (71.5122, 6.2675) centre (71.5122, 6.4263) ccw
  arc A1030 (80.398, 5.7976) -> (80.398, 5.4801) centre (80.398, 5.6389) ccw
  arc A1031 (81.8099, 5.7609) -> (81.6883, 6.0542) centre (81.7491, 5.9076) ccw
  line L166 (72.7502, 6.4041) -> (73.2468, 5.9076)
  arc A1032 (83.8136, 11.3225) -> (83.4961, 11.3225) centre (83.6548, 11.3225) ccw
  line L167 (73.8956, 5.6388) -> (74.5979, 5.6388)
  arc A1033 (75.5966, 6.4649) -> (75.89, 6.3434) centre (75.7433, 6.4041) ccw
  arc A1034 (73.8348, 5.4921) -> (73.9563, 5.7855) centre (73.8956, 5.6388) ccw
  arc A1035 (1.2746, 35.0709) -> (0.9812, 35.1924) centre (1.1279, 35.1316) ccw
  line L168 (71.5122, 6.4262) -> (72.7411, 6.4262)
  line L169 (82.5144, 7.053) -> (82.5144, 7.7552)
  arc A1036 (75.7524, 6.585) -> (75.7524, 6.2675) centre (75.7524, 6.4263) ccw
  arc A1037 (73.3075, 6.0542) -> (73.186, 5.7609) centre (73.2468, 5.9076) ccw
  arc A1038 (0.7429, 33.9944) -> (1.0605, 33.9944) centre (0.9017, 33.9944) ccw
  arc A1039 (82.6611, 6.9922) -> (82.3678, 7.1137) centre (82.5145, 7.053) ccw
  arc A1040 (71.4515, 6.2795) -> (71.573, 6.5729) centre (71.5122, 6.4262) ccw
  arc A1041 (73.8956, 5.7976) -> (73.8956, 5.4801) centre (73.8956, 5.6389) ccw
  arc A1042 (75.1344, 6.0198) -> (75.359, 5.7953) centre (75.2467, 5.9075) ccw
  arc A1043 (79.1059, 6.3434) -> (79.3993, 6.4649) centre (79.2526, 6.4041) ccw
  arc A1044 (68.1051, 9.3408) -> (68.1051, 9.0234) centre (68.1051, 9.1821) ccw
  arc A1045 (6.6867, 33.177) -> (6.5652, 32.8836) centre (6.626, 33.0303) ccw
  arc A1046 (84.2752, 11.7183) -> (84.0506, 11.9428) centre (84.1629, 11.8305) ccw
  arc A1047 (57.0464, 19.8168) -> (56.8218, 19.5923) centre (56.9341, 19.7046) ccw
  arc A1048 (57.6923, 18.7218) -> (57.9168, 18.9464) centre (57.8045, 18.8341) ccw
  line L170 (83.2309, 8.5029) -> (83.506, 8.778)
  arc A1049 (82.652, 7.8381) -> (82.3586, 7.7165) centre (82.5053, 7.7773) ccw
  arc A1050 (60.0646, 20.9355) -> (59.7471, 20.9355) centre (59.9059, 20.9355) ccw
  line L171 (57.8045, 21.8059) -> (56.9341, 20.9355)
  line L172 (4.004, 35.7759) -> (2.092, 35.7759)
  line L173 (82.5053, 7.7773) -> (83.2309, 8.5029)
  arc A1051 (59.1477, 21.9182) -> (58.9232, 21.6936) centre (59.0355, 21.8059) ccw
  arc A1052 (1.0484, 34.0552) -> (0.755, 33.9337) centre (0.9017, 33.9945) ccw
  arc A1053 (82.3557, 7.053) -> (82.6732, 7.053) centre (82.5145, 7.053) ccw
  line L174 (83.506, 8.778) -> (83.6549, 9.1374)
  arc A1054 (57.8045, 21.9646) -> (57.8045, 21.6471) centre (57.8045, 21.8059) ccw
  arc A1055 (83.3432, 8.3907) -> (83.1187, 8.6152) centre (83.231, 8.5029) ccw
  arc A1056 (59.0355, 18.6753) -> (59.0355, 18.9929) centre (59.0355, 18.8341) ccw
  arc A1057 (57.0928, 20.9355) -> (56.7754, 20.9355) centre (56.9341, 20.9355) ccw
  line L175 (82.5144, 7.7552) -> (82.5053, 7.7773)
  arc A1058 (1.6582, 35.4374) -> (1.4336, 35.6619) centre (1.5459, 35.5496) ccw
  arc A1059 (2.092, 35.9346) -> (2.092, 35.6171) centre (2.092, 35.7759) ccw
  arc A1060 (1.0157, 35.2439) -> (1.2402, 35.0194) centre (1.1279, 35.1317) ccw
  arc A1061 (0.9812, 33.3876) -> (1.2746, 33.5091) centre (1.1279, 33.4484) ccw
  arc A1062 (83.3594, 8.8388) -> (83.6527, 8.7173) centre (83.5061, 8.7781) ccw
  line L176 (59.0355, 18.8341) -> (59.9059, 19.7045)
  arc A1063 (0.755, 34.6463) -> (1.0484, 34.5248) centre (0.9017, 34.5855) ccw
  arc A1064 (83.5426, 11.4348) -> (83.7672, 11.2103) centre (83.6549, 11.3225) ccw
  line L177 (83.6549, 9.1374) -> (83.6549, 11.3225)
  arc A1065 (83.4961, 9.1374) -> (83.8136, 9.1374) centre (83.6548, 9.1374) ccw
  arc A1066 (57.8045, 18.9929) -> (57.8045, 18.6753) centre (57.8045, 18.8341) ccw
  arc A1067 (82.099, 6.4649) -> (82.3924, 6.3434) centre (82.2457, 6.4042) ccw
  arc A1068 (82.393, 7.8896) -> (82.6175, 7.665) centre (82.5053, 7.7773) ccw
  arc A1069 (4.004, 35.6171) -> (4.004, 35.9346) centre (4.004, 35.7759) ccw
  arc A1070 (1.4852, 35.6963) -> (1.6067, 35.403) centre (1.5459, 35.5496) ccw
  arc A1071 (83.1187, 8.6152) -> (83.3432, 8.3907) centre (83.231, 8.503) ccw
  line L178 (2.092, 35.7759) -> (1.5459, 35.5497)
  arc A1072 (58.9232, 18.9464) -> (59.1477, 18.7218) centre (59.0355, 18.8341) ccw
  arc A1073 (82.3678, 7.6945) -> (82.6611, 7.816) centre (82.5145, 7.7553) ccw
  line L179 (59.9059, 19.7045) -> (59.9059, 20.9355)
  line L180 (59.0355, 21.8059) -> (57.8045, 21.8059)
  line L181 (56.9341, 20.9355) -> (56.9341, 19.7045)
  arc A1074 (2.1528, 35.6292) -> (2.0313, 35.9226) centre (2.092, 35.7759) ccw
  arc A1075 (57.9168, 21.6936) -> (57.6923, 21.9182) centre (57.8046, 21.8059) ccw
  arc A1076 (56.8218, 21.0477) -> (57.0464, 20.8232) centre (56.9341, 20.9354) ccw
  line L182 (56.9341, 19.7045) -> (57.8045, 18.8341)
  line L183 (1.5459, 35.5497) -> (1.1279, 35.1317)
  line L184 (59.9059, 20.9355) -> (59.0355, 21.8059)
  arc A1077 (17.4808, 44.6377) -> (17.7053, 44.8622) centre (17.593, 44.7499) ccw
  arc A1078 (56.7754, 19.7045) -> (57.0928, 19.7045) centre (56.9341, 19.7045) ccw
  arc A1079 (83.6183, 8.6658) -> (83.3938, 8.8903) centre (83.5061, 8.7781) ccw
  arc A1080 (83.8016, 9.0767) -> (83.5082, 9.1982) centre (83.6549, 9.1374) ccw
  arc A1081 (59.0355, 21.6471) -> (59.0355, 21.9646) centre (59.0355, 21.8059) ccw
  arc A1082 (59.7471, 19.7045) -> (60.0646, 19.7045) centre (59.9059, 19.7045) ccw
  arc A1083 (17.8886, 31.7487) -> (17.5952, 31.8702) centre (17.7419, 31.8095) ccw
  line L185 (4.5501, 33.0303) -> (4.8319, 33.3121)
  arc A1084 (82.6732, 7.7552) -> (82.3557, 7.7552) centre (82.5145, 7.7552) ccw
  arc A1085 (3.9432, 32.9508) -> (4.0647, 32.6574) centre (4.004, 32.8041) ccw
  line L186 (83.6549, 11.3225) -> (84.1629, 11.8305)
  line L187 (57.8045, 18.8341) -> (59.0355, 18.8341)
  line L188 (2.092, 32.8041) -> (4.004, 32.8041)
  arc A1086 (12.5878, 29.7976) -> (12.4663, 29.5043) centre (12.5271, 29.651) ccw
  arc A1087 (4.4378, 33.1426) -> (4.6623, 32.9181) centre (4.55, 33.0304) ccw
  arc A1088 (15.8547, 29.5043) -> (15.7332, 29.7976) centre (15.7939, 29.651) ccw
  arc A1089 (15.3738, 29.6488) -> (15.4953, 29.3554) centre (15.4345, 29.5021) ccw
  arc A1090 (4.6108, 32.8836) -> (4.4893, 33.177) centre (4.5501, 33.0303) ccw
  line L189 (17.593, 31.4501) -> (17.7419, 31.8095)
  arc A1091 (9.0232, 32.9508) -> (9.1447, 32.6574) centre (9.084, 32.8041) ccw
  arc A1092 (15.6817, 29.7632) -> (15.9062, 29.5387) centre (15.794, 29.651) ccw
  line L190 (12.8865, 29.5021) -> (15.4345, 29.5021)
  arc A1093 (9.084, 32.6454) -> (9.084, 32.9628) centre (9.084, 32.8041) ccw
  line L191 (12.5271, 29.651) -> (12.8865, 29.5021)
  arc A1094 (17.5831, 31.8095) -> (17.9006, 31.8095) centre (17.7419, 31.8095) ccw
  arc A1095 (17.4464, 31.5108) -> (17.7397, 31.3893) centre (17.5931, 31.4501) ccw
  line L192 (17.3179, 45.025) -> (15.1096, 47.2333)
  arc A1096 (6.3441, 33.1534) -> (6.3441, 33.4708) centre (6.3441, 33.3121) ccw
  arc A1097 (9.3498, 32.7424) -> (9.2283, 33.0357) centre (9.2891, 32.8891) ccw
  line L193 (1.1279, 33.4483) -> (1.5459, 33.0303)
  arc A1098 (6.5136, 32.9181) -> (6.7382, 33.1426) centre (6.6259, 33.0304) ccw
  arc A1099 (15.2219, 47.3456) -> (14.9974, 47.1211) centre (15.1097, 47.2334) ccw
  line L194 (15.1096, 47.2333) -> (15.24, 47.3637)
  arc A1100 (17.7397, 44.8107) -> (17.4464, 44.6892) centre (17.5931, 44.7499) ccw
  line L195 (17.593, 44.7499) -> (17.3179, 45.025)
  arc A1101 (19.9142, 47.1562) -> (19.77, 47.4391) centre (19.8421, 47.2977) ccw
  arc A1102 (17.4302, 45.1373) -> (17.2057, 44.9128) centre (17.318, 45.025) ccw
  line L196 (1.5459, 33.0303) -> (2.092, 32.8041)
  arc A1103 (20.1279, 47.309) -> (19.9412, 47.5659) centre (20.0346, 47.4375) ccw
  line L197 (17.7419, 31.8095) -> (17.7419, 44.3905)
  arc A1104 (1.6067, 33.177) -> (1.4852, 32.8836) centre (1.546, 33.0303) ccw
  arc A1105 (4.004, 32.6454) -> (4.004, 32.9628) centre (4.004, 32.8041) ccw
  line L198 (9.084, 32.8041) -> (9.289, 32.889)
  arc A1106 (7.172, 32.9628) -> (7.172, 32.6454) centre (7.172, 32.8041) ccw
  arc A1107 (4.9441, 33.1998) -> (4.7196, 33.4244) centre (4.8319, 33.3121) ccw
  line L199 (4.8319, 33.3121) -> (6.3441, 33.3121)
  arc A1108 (17.2057, 44.9128) -> (17.4302, 45.1373) centre (17.3179, 45.0251) ccw
  arc A1109 (1.2402, 33.5606) -> (1.0157, 33.336) centre (1.128, 33.4483) ccw
  arc A1110 (15.3523, 47.2514) -> (15.1277, 47.4759) centre (15.24, 47.3636) ccw
  arc A1111 (12.8257, 29.3554) -> (12.9472, 29.6488) centre (12.8865, 29.5021) ccw
  line L200 (17.7419, 44.3905) -> (17.593, 44.7499)
  line L201 (6.3441, 33.3121) -> (6.6259, 33.0303)
  arc A1112 (12.8865, 29.6609) -> (12.8865, 29.3434) centre (12.8865, 29.5022) ccw
  line L202 (15.24, 47.3637) -> (15.51, 47.0937)
  arc A1113 (9.4013, 33.0013) -> (9.1768, 32.7768) centre (9.2891, 32.8891) ccw
  line L203 (7.172, 32.8041) -> (9.084, 32.8041)
  arc A1114 (7.1113, 32.6574) -> (7.2328, 32.9508) centre (7.1721, 32.8041) ccw
  arc A1115 (15.4345, 29.3434) -> (15.4345, 29.6609) centre (15.4345, 29.5022) ccw
  arc A1116 (6.4564, 33.4244) -> (6.2319, 33.1998) centre (6.3442, 33.3121) ccw
  arc A1117 (1.4336, 32.9181) -> (1.6582, 33.1426) centre (1.5459, 33.0304) ccw
  arc A1118 (12.4148, 29.5387) -> (12.6393, 29.7632) centre (12.5271, 29.651) ccw
  arc A1119 (17.7053, 31.3378) -> (17.4808, 31.5623) centre (17.593, 31.4501) ccw
  line L204 (15.4345, 29.5021) -> (15.7939, 29.651)
  line L205 (4.004, 32.8041) -> (4.5501, 33.0303)
  line L206 (6.6259, 33.0303) -> (7.172, 32.8041)
  arc A1120 (2.0313, 32.6574) -> (2.1528, 32.9508) centre (2.0921, 32.8041) ccw
  arc A1121 (4.8319, 33.4708) -> (4.8319, 33.1534) centre (4.8319, 33.3121) ccw
  arc A1122 (2.092, 32.9628) -> (2.092, 32.6454) centre (2.092, 32.8041) ccw
  line L207 (15.7939, 29.651) -> (17.593, 31.4501)
  arc A1123 (17.9006, 44.3905) -> (17.5831, 44.3905) centre (17.7419, 44.3905) ccw
  arc A1124 (17.5952, 44.3298) -> (17.8886, 44.4513) centre (17.7419, 44.3905) ccw
  arc A1125 (14.9974, 47.3456) -> (15.2219, 47.1211) centre (15.1097, 47.2334) ccw
  line L208 (9.289, 32.889) -> (12.5271, 29.651)